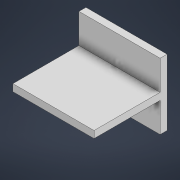
# Autodesk Inventor part: Fof
Saved by Autodesk Inventor 2022 (Build 260153000, 153)
## iProperties
Created: 2023-05-09
Part Number: Fof
Material: Generic
Document SubType Name: Modeling
Designer: Jakob Saugbjerg
Density: 1 g/cm^3
Appearance: Default
Author: Jakob Saugbjerg
Autodesk Inventor part; units mm, degrees
ref_plane "YZ Plane" through (0, 0, 0) normal (1, 0, 0) x (0, 1, 0)
ref_plane "XZ Plane" through (0, 0, 0) normal (0, 1, 0) x (-1, 0, 0)
ref_plane "XY Plane" through (0, 0, 0) normal (0, 0, 1) x (1, 0, 0)
sketch "Sketch1" plane through (0, 0, 0) normal (0, 0, 1) x (1, 0, 0)
  line L0 (0, 0) -> (35, 0)
  line L1 (35, 0) -> (35, 28.5)
  line L2 (35, 28.5) -> (0, 28.5)
  line L3 (0, 28.5) -> (0, 0)
  dimension "d0" = 35
  dimension "d1" = 28.5
  constraints: 8 end point, 2 parallel, 1 horizontal, 1 perpendicular
  measures "d0" distance of L2.end L1.end
  measures "d1" distance of L1.end L0.end
extrude "Extrusion1" add sketch "Sketch1" along normal blind 3
sketch "Sketch2" plane through (0, 0, 3) normal (0, 0, 1) x (1, 0, 0)
  line L0 (35, 0) -> (35, 28.5) projected
  line L1 (0, 12.75) -> (35, 12.75)
  line L2 (35, 12.75) -> (35, 15.75)
  line L3 (35, 15.75) -> (0, 15.75)
  line L4 (0, 15.75) -> (0, 12.75)
  line L5 (0, 12.75) -> (35, 15.75) construction
  line L6 (35, 12.75) -> (0, 15.75) construction
  point P0 (0, 0)
  point P1 (17.5, 14.25)
  dimension "d4" = 3
  constraints: 12 end point, 2 midpoint, 2 parallel, 1 horizontal, 1 perpendicular, 1 point on line
  measures "d4" distance of L2.end L1.end
extrude "Extrusion2" add sketch "Sketch2" along normal blind 28.5
body "Solid1"
